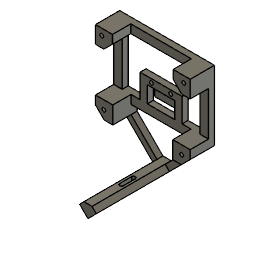
土台1(new) (Autodesk Fusion 360 design; units mm, degrees)
Autodesk Fusion 360 part; units mm, degrees
sketch "スケッチ1" plane through (0, 0, 0) normal (0, 0, 1) x (1, 0, 0)
  line L0 (-38.8909, 38.8909) -> (0, 0)
  line L1 (0, 0) -> (38.8909, 38.8909)
  line L2 (38.8909, 38.8909) -> (-38.8909, 38.8909) construction
  line L3 (0, 38.8909) -> (0, 0) construction
  line L4 (-24.5921, 31.6632) -> (-3.3789, 10.45)
  line L5 (-3.3789, 10.45) -> (3.3789, 10.45)
  line L6 (3.3789, 10.45) -> (24.5921, 31.6632)
  line L7 (24.5921, 31.6632) -> (24.5921, 38.8909)
  line L8 (-24.5921, 38.8909) -> (-24.5921, 31.6632)
  line L9 (-24.5921, 38.8909) -> (24.5921, 38.8909)
  line L10 (-38.8909, 38.8909) -> (-38.8909, 45.9909)
  line L11 (-31.8909, 45.9909) -> (31.8909, 45.9909)
  line L12 (38.8909, 45.9909) -> (38.8909, 38.8909)
  line L13 (31.8909, 45.9909) -> (-31.8909, 45.9909)
  line L14 (-38.8909, 45.9909) -> (-38.8909, 95.9909)
  line L15 (-38.8909, 95.9909) -> (38.8909, 95.9909)
  line L16 (38.8909, 95.9909) -> (38.8909, 45.9909)
  line L17 (38.8909, 45.9909) -> (-38.8909, 95.9909) construction
  line L18 (-38.8909, 45.9909) -> (38.8909, 95.9909) construction
  line L19 (-31.8909, 45.9909) -> (-31.8909, 81.9198)
  line L20 (-24.8198, 88.9909) -> (24.8198, 88.9909)
  line L21 (31.8909, 81.9198) -> (31.8909, 45.9909)
  line L22 (-24.8198, 88.9909) -> (-31.8909, 81.9198)
  line L23 (24.8198, 88.9909) -> (31.8909, 81.9198)
  point P0 (0, 70.9909)
  point P1 (0, 70.9909)
  dimension "d1" = 55
  dimension "d3" = 55
  dimension "d4" = 5
  dimension "d5" = 5
  dimension "d6" = 30
  dimension "d7" = 30
  dimension "d8" = 10.45
  dimension "d9" = 7.1
  dimension "d10" = 50
  dimension "d11" = 7
  dimension "d13" = 45
  dimension "d14" = 45
  dimension "d15" = 10
  dimension "d16" = 10
  dimension "d17" = 7
  dimension "d18" = 7
  dimension "d19" = 57.1
  dimension "d20" = 7.1
  constraint coincident L0.end L1.start
  constraint horizontal L2
  constraint midpoint L2 L3.start
  constraint perpendicular L3 L5
  constraint parallel L0 L4
  constraint parallel L1 L6
  constraint perpendicular L0 L1
  constraint vertical L8
  constraint vertical L7
  constraint coincident L2 L8.start
  constraint coincident L2 L7.end
  constraint coincident L0.start L2.end
  constraint horizontal L11
  constraint vertical L10
  constraint vertical L12
  constraint horizontal L13
  constraint perpendicular L13 L14
  constraint parallel L13 L15
  constraint parallel L14 L16
  constraint coincident L17 P1
  constraint coincident L18 P1
  constraint coincident L10.end L14.start
  constraint coincident P1 P0
  measures "d1" distance of L0.end L1.end
  measures "d3" distance of L0.start L0.end
  measures "d4" distance of L1 L6
  measures "d5" distance of L0 L4
  measures "d6" distance of L5.end L6.end
  measures "d7" distance of L4.start L4.end
  measures "d8" distance of L0.end L5
  measures "d9" distance of L9 L11
  measures "d10" distance of L12.start L15.end
  measures "d11" distance of L16 L21
  measures "d13" angle of L20 L22
  measures "d14" angle of L20 L23
  measures "d15" distance of L20.start L19.end
  measures "d16" distance of L20.end L21.start
  measures "d17" distance of L15 L20
  measures "d18" distance of L14 L19
  measures "d19" distance of L9 L15
  measures "d20" distance of L0.start L10.end
extrude "押し出し1" add sketch "スケッチ1" along normal mid plane 5 makes body 1
sketch "スケッチ2" plane through (0, 0, 2.5) normal (0, 0, 1) x (1, 0, 0)
  line L0 (-31.8909, 81.9198) -> (-24.8198, 88.9909)
  line L1 (-24.8198, 88.9909) -> (24.8198, 88.9909)
  line L2 (24.8198, 88.9909) -> (31.8909, 81.9198)
  line L3 (31.8909, 81.9198) -> (31.8909, 45.9909)
  line L4 (31.8909, 45.9909) -> (-31.8909, 45.9909)
  line L5 (-31.8909, 45.9909) -> (-31.8909, 81.9198)
  line L6 (-3.3789, 10.45) -> (-24.5921, 31.6632)
  line L7 (-24.5921, 31.6632) -> (-24.5921, 38.8909)
  line L8 (-24.5921, 38.8909) -> (24.5921, 38.8909)
  line L9 (24.5921, 38.8909) -> (24.5921, 31.6632)
  line L10 (24.5921, 31.6632) -> (3.3789, 10.45)
  line L11 (3.3789, 10.45) -> (-3.3789, 10.45)
  line L12 (-38.8909, 38.8909) -> (0, 0)
  line L13 (0, 0) -> (38.8909, 38.8909)
  line L14 (38.8909, 38.8909) -> (38.8909, 95.9909)
  line L15 (38.8909, 95.9909) -> (-38.8909, 95.9909)
  line L16 (-38.8909, 95.9909) -> (-38.8909, 38.8909)
  line L17 (-24.8198, 95.9909) -> (-24.8198, 88.9909)
  line L18 (-24.8198, 88.9909) -> (-31.8909, 81.9198)
  line L19 (-31.8909, 81.9198) -> (-38.8909, 81.9198)
  line L20 (-38.8909, 81.9198) -> (-38.8909, 95.9909)
  line L21 (-38.8909, 95.9909) -> (-24.8198, 95.9909)
  line L22 (24.8198, 95.9909) -> (24.8198, 88.9909)
  line L23 (24.8198, 88.9909) -> (31.8909, 81.9198)
  line L24 (31.8909, 81.9198) -> (38.8909, 81.9198)
  line L25 (38.8909, 81.9198) -> (38.8909, 95.9909)
  line L26 (38.8909, 95.9909) -> (24.8198, 95.9909)
  line L27 (-24.5921, 45.9909) -> (-24.5921, 31.6632)
  line L28 (-24.5921, 31.6632) -> (-31.6632, 31.6632)
  line L29 (-31.6632, 31.6632) -> (-38.8909, 38.8909)
  line L30 (-38.8909, 38.8909) -> (-38.8909, 45.9909)
  line L31 (-38.8909, 45.9909) -> (-24.5921, 45.9909)
  line L32 (24.5921, 45.9909) -> (24.5921, 31.6632)
  line L33 (24.5921, 31.6632) -> (31.6632, 31.6632)
  line L34 (31.6632, 31.6632) -> (38.8909, 38.8909)
  line L35 (38.8909, 38.8909) -> (38.8909, 45.9909)
  line L36 (38.8909, 45.9909) -> (24.5921, 45.9909)
  line L37 (-3.3789, 10.45) -> (-6.9145, 6.9145)
  line L38 (-6.9145, 6.9145) -> (0, 0)
  line L39 (0, 0) -> (6.9145, 6.9145)
  line L40 (6.9145, 6.9145) -> (3.3789, 10.45)
  line L41 (3.3789, 10.45) -> (-3.3789, 10.45)
  constraint coincident L15 L17.start
  constraint coincident L0.end L1.start
  constraint perpendicular L1 L17
  constraint coincident L0.start L5.end
  constraint coincident L16 L19.end
  constraint perpendicular L16 L19
  constraint coincident L15.end L16.start
  constraint coincident L15 L22.start
  constraint coincident L1.end L2.start
  constraint coincident L2.end L3.start
  constraint coincident L14 L24.end
  constraint perpendicular L14 L24
  constraint coincident L14.end L15.start
  constraint vertical L22
  constraint coincident L4 L27.start
  constraint coincident L6.end L7.start
  constraint coincident L12 L28.end
  constraint perpendicular L27 L28
  constraint vertical L27
  constraint coincident L16 L30.end
  constraint coincident L12.start L16.end
  constraint horizontal L31
  constraint vertical L32
  constraint perpendicular L32 L33
  constraint perpendicular L33 L35
  constraint coincident L4 L32.start
  constraint coincident L9.end L10.start
  constraint coincident L13 L33.end
  constraint coincident L14 L35.end
  constraint coincident L13.end L14.start
  constraint horizontal L36
  constraint coincident L6.start L11.end
  constraint coincident L12 L37.end
  constraint perpendicular L12 L37
  constraint perpendicular L12 L39
  constraint coincident L10.end L11.start
  constraint coincident L13 L39.end
  constraint coincident L12.end L13.start
  constraint perpendicular L13 L40
extrude "押し出し2" add sketch "スケッチ2" along normal blind 15 contours L0 L15 L16 L17 L18 L19 L20 L21 | L4 L7 L12 L16 L27 L28 L29 L30 L31 | L2 L14 L15 L22 L23 L24 L25 L26 | L4 L9 L13 L14 L32 L33 L34 L35 L36 bodies 1
extrude "押し出し3" add sketch "スケッチ2" along normal blind 60 contours L11 L12 L13 L37 L38 L39 L40 L41 bodies 1
sketch "スケッチ3" plane through (0, 0, -2.5) normal (0, 0, -1) x (-1, 0, 0)
  line L0 (24.8198, 88.9909) -> (31.8909, 81.9198)
  line L1 (31.8909, 81.9198) -> (31.8909, 45.9909)
  line L2 (31.8909, 45.9909) -> (-31.8909, 45.9909)
  line L3 (-31.8909, 45.9909) -> (-31.8909, 81.9198)
  line L4 (-31.8909, 81.9198) -> (-24.8198, 88.9909)
  line L5 (-24.8198, 88.9909) -> (24.8198, 88.9909)
  line L6 (24.5921, 31.6632) -> (3.3789, 10.45)
  line L7 (3.3789, 10.45) -> (-3.3789, 10.45)
  line L8 (-3.3789, 10.45) -> (-24.5921, 31.6632)
  line L9 (-24.5921, 31.6632) -> (-24.5921, 38.8909)
  line L10 (-24.5921, 38.8909) -> (24.5921, 38.8909)
  line L11 (24.5921, 38.8909) -> (24.5921, 31.6632)
  line L12 (0, 0) -> (38.8909, 38.8909)
  line L13 (38.8909, 38.8909) -> (38.8909, 95.9909)
  line L14 (38.8909, 95.9909) -> (-38.8909, 95.9909)
  line L15 (-38.8909, 95.9909) -> (-38.8909, 38.8909)
  line L16 (-38.8909, 38.8909) -> (0, 0)
  line L17 (-38.8909, 95.9909) -> (-28.3553, 85.4553) construction
  line L18 (38.8909, 95.9909) -> (28.3553, 85.4553) construction
  circle A0 centre (-33.6231, 90.7231) radius 3.25
  circle A1 centre (33.6231, 90.7231) radius 3.25
  circle A2 centre (-31.8909, 38.8909) radius 3.25
  circle A3 centre (31.8909, 38.8909) radius 3.25
  line L19 (-24.5921, 38.8909) -> (-38.8909, 38.8909) construction
  line L20 (-31.8909, 45.9909) -> (-31.8909, 31.8909) construction
  line L21 (24.5921, 38.8909) -> (38.8909, 38.8909) construction
  line L22 (31.8909, 45.9909) -> (31.8909, 31.8909) construction
  circle A4 centre (-31.8909, 38.8909) radius 1.5
  circle A5 centre (31.8909, 38.8909) radius 1.5
  circle A6 centre (33.6231, 90.7231) radius 1.5
  circle A7 centre (-33.6231, 90.7231) radius 1.5
  dimension "d27" = 6.5
  dimension "d28" = 6.5
  dimension "d29" = 6.5
  dimension "d30" = 6.5
  dimension "d31" = 3
  dimension "d32" = 3
  dimension "d33" = 3
  dimension "d34" = 3
  constraint coincident L14.end L15.start
  constraint midpoint L4 L17.end
  constraint coincident L13.end L14.start
  constraint midpoint L0 L18.end
  constraint midpoint L17 A0.centre
  constraint midpoint L18 A1.centre
  constraint coincident L9.end L10.start
  constraint coincident L15.end L16.start
  constraint coincident L2.end L3.start
  constraint coincident L16 L20.end
  constraint perpendicular L19 L20
  constraint coincident A2.centre L19
  constraint coincident A2.centre L20
  constraint coincident L10.end L11.start
  constraint coincident L12.end L13.start
  constraint coincident L1.end L2.start
  constraint coincident L12 L22.end
  constraint perpendicular L21 L22
  constraint coincident A3.centre L22
  constraint coincident A3.centre L21
  constraint concentric A2 A4
  constraint concentric A3 A5
  constraint concentric A1 A6
  constraint concentric A0 A7
  measures "d27" diameter of A0
  measures "d28" diameter of A1
  measures "d29" diameter of A2
  measures "d30" diameter of A3
  measures "d31" diameter of A4
  measures "d32" diameter of A5
  measures "d33" diameter of A6
  measures "d34" diameter of A7
extrude "押し出し4" cut sketch "スケッチ3" against normal blind 25 contours A4 | A5 | A6 | A7 bodies 1
extrude "押し出し5" cut sketch "スケッチ3" against normal blind 15 contours A0 | A1 | A2 | A3 bodies 1
sketch "スケッチ4" plane through (0, 10.45, 0) normal (0, 1, 0) x (-1, 0, 0)
  line L0 (3.3789, -2.5) -> (3.3789, 2.5)
  line L1 (3.3789, 2.5) -> (3.3789, 62.5)
  line L2 (3.3789, 62.5) -> (-3.3789, 62.5)
  line L3 (-3.3789, 62.5) -> (-3.3789, 2.5)
  line L4 (-3.3789, 2.5) -> (-3.3789, -2.5)
  line L5 (-3.3789, -2.5) -> (3.3789, -2.5)
  arc A0 (1.5, 35) -> (-1.5, 35) centre (0, 35) ccw
  arc A1 (-1.5, 25) -> (1.5, 25) centre (0, 25) ccw
  line L6 (0, 35) -> (0, 25) construction
  line L7 (-1.5, 35) -> (-1.5, 25)
  line L8 (1.5, 35) -> (1.5, 25)
  line L9 (0, 25) -> (0, 0) construction
  dimension "d39" = 1.5
  dimension "d40" = 1.5
  dimension "d41" = 25
  dimension "d42" = 35
  constraint coincident A0.centre L6.start
  constraint coincident A1.centre L6.end
  constraint tangent A1 L8
  constraint tangent A1 L7
  constraint tangent A0 L7
  constraint coincident A1.start L7.end
  constraint vertical L7
  constraint coincident L9.end origin
  constraint vertical L9
  constraint tangent A0 L8
  measures "d39" radius of A0
  measures "d40" radius of A1
  measures "d41" vertical distance of L9.end A1.centre
  measures "d42" vertical distance of L9.end A0.centre
extrude "押し出し6" cut sketch "スケッチ4" against normal blind 4 contours A0 A1 L7 L8 bodies 1
sketch "スケッチ5" plane through (0, 0, -2.5) normal (0, 0, -1) x (-1, 0, 0)
  line L0 (24.8198, 88.9909) -> (31.8909, 81.9198)
  line L1 (31.8909, 81.9198) -> (31.8909, 45.9909)
  line L2 (31.8909, 45.9909) -> (-31.8909, 45.9909)
  line L3 (-31.8909, 45.9909) -> (-31.8909, 81.9198)
  line L4 (-31.8909, 81.9198) -> (-24.8198, 88.9909)
  line L5 (-24.8198, 88.9909) -> (24.8198, 88.9909)
  line L6 (24.5921, 31.6632) -> (3.3789, 10.45)
  line L7 (3.3789, 10.45) -> (-3.3789, 10.45)
  line L8 (-3.3789, 10.45) -> (-24.5921, 31.6632)
  line L9 (-24.5921, 31.6632) -> (-24.5921, 38.8909)
  line L10 (-24.5921, 38.8909) -> (24.5921, 38.8909)
  line L11 (24.5921, 38.8909) -> (24.5921, 31.6632)
  line L12 (0, 0) -> (38.8909, 38.8909)
  line L13 (38.8909, 38.8909) -> (38.8909, 95.9909)
  line L14 (38.8909, 95.9909) -> (-38.8909, 95.9909)
  line L15 (-38.8909, 95.9909) -> (-38.8909, 38.8909)
  line L16 (-38.8909, 38.8909) -> (0, 0)
  circle A0 centre (31.8909, 38.8909) radius 3.25
  circle A1 centre (-33.6231, 90.7231) radius 3.25
  circle A2 centre (33.6231, 90.7231) radius 3.25
  circle A3 centre (-31.8909, 38.8909) radius 3.25
  line L17 (-11.25, 45.9909) -> (-11.25, 59.4909)
  line L18 (-11.25, 59.4909) -> (11.25, 59.4909)
  line L19 (11.25, 59.4909) -> (11.25, 45.9909)
  line L20 (-17.25, 45.9909) -> (-17.25, 65.4909)
  line L21 (-17.25, 65.4909) -> (17.25, 65.4909)
  line L22 (17.25, 65.4909) -> (17.25, 45.9909)
  line L23 (0, 0) -> (0, 59.4909) construction
  circle A4 centre (-7.9, 62.4909) radius 1.5
  circle A5 centre (7.9, 62.4909) radius 1.5
  line L24 (-7.9, 62.4909) -> (7.9, 62.4909) construction
  line L25 (0, 59.4909) -> (0, 62.4909) construction
  dimension "d45" = 6
  dimension "d46" = 6
  dimension "d47" = 6
  dimension "d48" = 22.5
  dimension "d49" = 13.5
  dimension "d50" = 15.8
  dimension "d51" = 3
  dimension "d52" = 3
  dimension "d53" = 3
  constraint coincident L2 L17.start
  constraint coincident L2 L19.end
  constraint vertical L19
  constraint horizontal L18
  constraint vertical L17
  constraint coincident L2 L20.start
  constraint perpendicular L2 L20
  constraint perpendicular L20 L21
  constraint coincident L2 L22.end
  constraint perpendicular L2 L22
  constraint coincident L12.start L16.end
  constraint coincident L18 L23.end
  constraint vertical L23
  constraint midpoint L18 L23.end
  constraint coincident A4.centre L24.start
  constraint coincident A5.centre L24.end
  constraint horizontal L24
  constraint coincident L24 L25.end
  constraint vertical L25
  constraint midpoint L24 L25.end
  measures "d45" distance of L18 L21
  measures "d46" distance of L19 L22
  measures "d47" distance of L17 L20
  measures "d48" distance of L17.end L18.end
  measures "d49" distance of L17.start L17.end
  measures "d50" distance of A4.centre A5.centre
  measures "d51" distance of L23.end L25.end
  measures "d52" diameter of A4
  measures "d53" diameter of A5
extrude "押し出し7" add sketch "スケッチ5" against normal blind 5 contours L2 L17 L18 L19 L20 L21 L22 bodies 1
sketch "スケッチ6" plane through (0, 0, -2.5) normal (0, 0, -1) x (-1, 0, 0)
  line L0 (11.25, 45.9909) -> (-11.25, 45.9909)
  line L1 (-11.25, 45.9909) -> (-11.25, 59.4909)
  line L2 (-11.25, 59.4909) -> (11.25, 59.4909)
  line L3 (11.25, 59.4909) -> (11.25, 45.9909)
  circle A0 centre (7.9, 62.4909) radius 1.5
  circle A1 centre (-7.9, 62.4909) radius 1.5
  line L4 (17.25, 45.9909) -> (17.25, 65.4909)
  line L5 (17.25, 65.4909) -> (-17.25, 65.4909)
  line L6 (-17.25, 65.4909) -> (-17.25, 45.9909)
  line L7 (-17.25, 45.9909) -> (-31.8909, 45.9909)
  line L8 (-31.8909, 45.9909) -> (-31.8909, 81.9198)
  line L9 (-31.8909, 81.9198) -> (-24.8198, 88.9909)
  line L10 (-24.8198, 88.9909) -> (24.8198, 88.9909)
  line L11 (24.8198, 88.9909) -> (31.8909, 81.9198)
  line L12 (31.8909, 81.9198) -> (31.8909, 45.9909)
  line L13 (31.8909, 45.9909) -> (17.25, 45.9909)
  line L14 (24.5921, 31.6632) -> (3.3789, 10.45)
  line L15 (3.3789, 10.45) -> (-3.3789, 10.45)
  line L16 (-3.3789, 10.45) -> (-24.5921, 31.6632)
  line L17 (-24.5921, 31.6632) -> (-24.5921, 38.8909)
  line L18 (-24.5921, 38.8909) -> (24.5921, 38.8909)
  line L19 (24.5921, 38.8909) -> (24.5921, 31.6632)
  line L20 (0, 0) -> (38.8909, 38.8909)
  line L21 (38.8909, 38.8909) -> (38.8909, 95.9909)
  line L22 (38.8909, 95.9909) -> (-38.8909, 95.9909)
  line L23 (-38.8909, 95.9909) -> (-38.8909, 38.8909)
  line L24 (-38.8909, 38.8909) -> (0, 0)
  circle A2 centre (31.8909, 38.8909) radius 3.25
  circle A3 centre (-33.6231, 90.7231) radius 3.25
  circle A4 centre (33.6231, 90.7231) radius 3.25
  circle A5 centre (-31.8909, 38.8909) radius 3.25
  line L25 (10.25, 64.4909) -> (-10.25, 64.4909)
  line L26 (-10.25, 64.4909) -> (-10.25, 49.0909)
  line L27 (-10.25, 49.0909) -> (10.25, 49.0909)
  line L28 (10.25, 49.0909) -> (10.25, 64.4909)
  line L29 (10.25, 64.4909) -> (-10.25, 49.0909) construction
  line L30 (-10.25, 64.4909) -> (10.25, 49.0909) construction
  line L31 (0, 56.7909) -> (0, 0) construction
  point P0 (0, 56.7909)
  dimension "d56" = 20.5
  dimension "d57" = 15.4
  dimension "d58" = 2
  constraint horizontal L25
  constraint perpendicular L25 L26
  constraint parallel L25 L27
  constraint parallel L26 L28
  constraint coincident L29 P0
  constraint coincident L30 P0
  constraint coincident P0 L31.start
  constraint coincident L20.start L24.end
  constraint perpendicular L15 L31
  measures "d56" distance of L25.start L25.end
  measures "d57" distance of L25.start L27.end
  measures "d58" distance of A0.centre L25
extrude "押し出し8" add sketch "スケッチ6" along normal blind 0.79 separate body contours L2 L26 L27 L28 | L2 L25 L26 L28 makes body 2
named bodies: "MPU6050"
